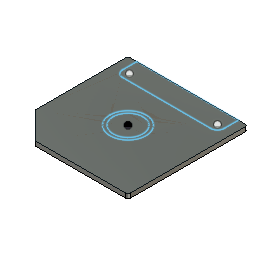
L_Floppy_Disk_v0 (Autodesk Fusion 360 design; units mm, degrees)
Autodesk Fusion 360 part; units mm, degrees
sketch "Sketch1" plane through (0, 0, 0) normal (0, 0, 1) x (1, 0, 0)
  line L0 (-64, 66.5) -> (64, 66.5)
  line L1 (66.5, 64) -> (66.5, -64)
  line L2 (64, -66.5) -> (-36.5, -66.5)
  line L3 (-66.5, -36.5) -> (-66.5, 64)
  line L4 (-36.5, -66.5) -> (-66.5, -36.5)
  arc A0 (-64, 66.5) -> (-66.5, 64) centre (-64, 64) ccw
  arc A1 (66.5, 64) -> (64, 66.5) centre (64, 64) ccw
  arc A2 (64, -66.5) -> (66.5, -64) centre (64, -64) ccw
extrude "Extrude1" add sketch "Sketch1" along normal blind 5
sketch "Sketch2" plane through (0, 0, 5) normal (0, 0, 1) x (-1, 0, 0)
  line L0 (36.5, 66.5) -> (-64, 66.5)
  arc A0 (-64, 66.5) -> (-66.5, 64) centre (-64, 64) ccw
  line L1 (-66.5, 64) -> (-66.5, -64)
  arc A1 (-66.5, -64) -> (-64, -66.5) centre (-64, -64) ccw
  line L2 (-64, -66.5) -> (64, -66.5)
  arc A2 (64, -66.5) -> (66.5, -64) centre (64, -64) ccw
  line L3 (66.5, -64) -> (66.5, 36.5)
  line L4 (66.5, 36.5) -> (36.5, 66.5)
  circle A3 centre (0, 0) radius 20
  circle A4 centre (0, 0) radius 16.5
  line L5 (-56.5, -66.5) -> (56.5, -66.5)
  line L6 (56.5, -66.5) -> (56.5, -50.5727)
  line L7 (49, -43.0727) -> (-49, -43.0727)
  line L8 (-56.5, -50.5727) -> (-56.5, -66.5)
  arc A5 (56.5, -50.5727) -> (49, -43.0727) centre (49, -50.5727) ccw
  arc A6 (-49, -43.0727) -> (-56.5, -50.5727) centre (-49, -50.5727) ccw
  constraint coincident A3.centre A4.centre
  constraint horizontal L5
  constraint equal A5 A6
